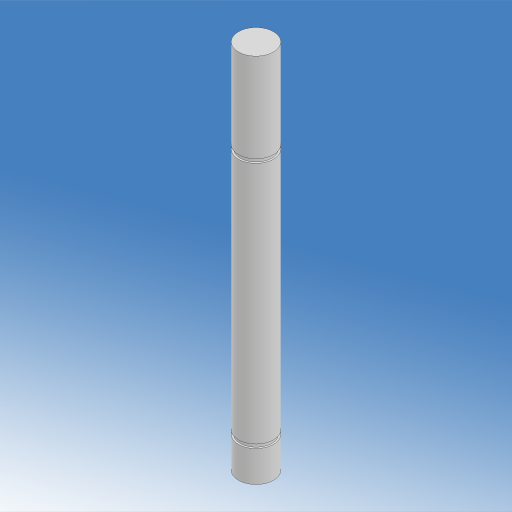
# Autodesk Inventor part: FlipperRoundShaft
Saved by Autodesk Inventor 2024 (Build 280153000, 153)
## iProperties
Created: 2024-02-06
Part Number: FlipperRoundShaft
Material: Generic
Document SubType Name: Modeling
Designer: seene
Density: 1 g/cm^3
Appearance: Default
Author: seene
Autodesk Inventor part; units mm, degrees
ref_plane "YZ Plane" through (0, 0, 0) normal (1, 0, 0) x (0, 1, 0)
ref_plane "XZ Plane" through (0, 0, 0) normal (0, 1, 0) x (-1, 0, 0)
sketch "Sketch1" plane through (0, 0, 0) normal (0, 1, 0) x (-1, 0, 0)
  circle A0 centre (0, 0) radius 4
  dimension "d0" = 8
  constraints: 1 centre point, 1 coincident
  measures "d0" diameter of A0
extrude "Extrusion1" add sketch "Sketch1" along normal blind 84.7
ref_plane "Work Plane2" through (0, 63.5, 0) normal (0, -1, 0) x (1, 0, 0)
ref_plane "Work Plane1" through (0, 8, 0) normal (0, -1, 0) x (1, 0, 0)
sketch "Sketch3" plane through (0, 0, 0) normal (0, 0, 1) x (1, 0, 0)
  line L0 (4, 84.7) -> (-4, 84.7) projected
  line L1 (4, 0) -> (-4, 0) projected
  line L2 (4, 84.7) -> (-4, 84.7) projected
  line L3 (4, 0) -> (-4, 0) projected
  line L4 (4, 63.5) -> (-4, 63.5)
  line L5 (3.6004, 63.5) -> (4.0004, 63.5)
  line L6 (4.0004, 63.5) -> (4.0004, 64.4)
  line L7 (4.0004, 64.4) -> (3.6004, 64.4)
  line L8 (3.6004, 64.4) -> (3.6004, 63.5)
  line L9 (0, -16.94) -> (0, 101.64) projected
  line L10 (-4, 8) -> (4.0004, 8)
  line L11 (4.0004, 8) -> (3.6004, 8)
  line L12 (3.6004, 8) -> (3.6004, 7.1)
  line L13 (3.6004, 7.1) -> (4.0004, 7.1)
  line L14 (4.0004, 7.1) -> (4.0004, 8)
  point P0 (0, 0)
  dimension "d7" = 63.5
  dimension "d8" = 0.4
  dimension "d9" = 0.9
  dimension "d12" = 8
  dimension "d13" = 0.4
  dimension "d14" = 0.9
  constraints: 20 end point, 4 horizontal, 4 parallel, 2 perpendicular, 1 point on line
  measures "d7" distance between parallel lines of L4 L1
  measures "d8" distance of L6.end L7.end
  measures "d9" distance of L7.end L5.start
  measures "d12" distance between parallel lines of L1 L10
  measures "d13" distance of L13.end L12.end
  measures "d14" distance of L12.end L11.end
revolve "Revolution2" cut sketch "Sketch3" angle 360 about axis through (0, -10, 0) along (0, 1, 0)
body "Solid1"
